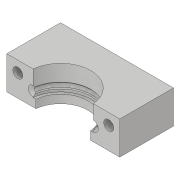
# Autodesk Inventor part: 7 peristaltic pump lid with lip2
Saved by Autodesk Inventor 2020 (Build 240168000, 168)
## iProperties
Created: 2018-08-21
Part Number: 7 peristaltic pump lid with lip2
Material: Generic
Document SubType Name: Modeling
Designer: mrbeh
Density: 1 g/cm^3
Appearance: Default
Author: mrbeh
Autodesk Inventor part; units mm, degrees
ref_plane "YZ Plane" through (0, 0, 0) normal (1, 0, 0) x (0, 1, 0)
ref_plane "XZ Plane" through (0, 0, 0) normal (0, 1, 0) x (-1, 0, 0)
sketch "Sketch1" plane through (0, 0, 0) normal (0, 1, 0) x (-1, 0, 0)
  line L0 (0, 0) -> (41, 0)
  line L1 (41, 0) -> (41, -41)
  line L2 (41, -41) -> (0, -41)
  line L3 (0, -41) -> (0, 0)
  dimension "d0" = 41
  dimension "d1" = 41
  constraints: 8 end point, 2 parallel, 1 horizontal, 1 perpendicular
  measures "d0" distance of L1.end L2.end
  measures "d1" distance of L0.end L1.end
extrude "Extrusion1" add sketch "Sketch1" along normal blind 9.5
sketch "Sketch3" plane through (0, 9.5, 0) normal (0, 1, 0) x (1, 0, 0)
  circle A0 centre (-20.5, 20.5) radius 10
  point P0 (0, 0)
  dimension "d5" = 20
  constraints: 1 centre point
  measures "d5" diameter of A0
extrude "Extrusion2" cut sketch "Sketch3" against normal blind 10
sketch "Sketch4" plane through (0, 9.5, 0) normal (0, 1, 0) x (1, 0, 0)
  circle A0 centre (-20.5, 20.5) radius 10 projected
  circle A1 centre (-20.5, 20.5) radius 11.75
  point P0 (0, 0)
  dimension "d8" = 23.5
  constraints: 1 centre point, 1 coincident
  measures "d8" diameter of A1
extrude "Extrusion3" cut sketch "Sketch4" against normal blind 5
sketch "Sketch5" plane through (0, 9.5, 0) normal (0, 1, 0) x (1, 0, 0)
  line L0 (-41, 41) -> (-41, 0) projected
  line L1 (-41, 0) -> (0, 0)
  line L2 (0, 0) -> (0, 41)
  line L3 (0, 41) -> (-41, 41)
  line L4 (-41, 41) -> (-41, 0)
  circle A0 centre (-20.5, 20.5) radius 11.75 projected
  circle A1 centre (-20.5, 20.5) radius 10
  constraints: 8 end point, 2 parallel, 1 centre point, 1 coincident, 1 horizontal, 1 perpendicular
extrude "Extrusion4" add sketch "Sketch5" along normal blind 4.5 contours L3 L2 L1 L0 | A0
sketch "Sketch6" plane through (-41, 0, 0) normal (0, 0, 1) x (1, 0, 0)
  line L0 (0, 0) -> (0, 14) projected
  line L1 (0, 14) -> (41, 14)
  line L2 (41, 14) -> (41, 0)
  line L3 (41, 0) -> (0, 0)
  line L4 (0, 0) -> (0, 14)
  constraints: 8 end point, 2 parallel, 1 horizontal, 1 perpendicular
extrude "Extrusion5" cut sketch "Sketch6" against normal blind 20.5
sketch "Sketch8" plane through (-41, 0, -20.5) normal (0, 0, 1) x (1, 0, 0)
  circle A0 centre (4, 10) radius 1.8
  point P0 (41, 0)
  dimension "d15" = 3.6
  constraints: 1 centre point
  measures "d15" diameter of A0
extrude "Extrusion6" cut sketch "Sketch8" against normal blind 20.5
ref_plane "Work Plane1" through (-20.5, 0, -41) normal (1, 0, 0) x (0, 0, -1)
mirror "Mirror1" about plane through (-20.5, 0, -41) normal (1, 0, 0) of "Extrusion6"
sketch "Sketch9" plane through (-41, 0, -20.5) normal (0, 0, 1) x (1, 0, 0)
  line L0 (10.5, 14) -> (10.5, 9.5) projected
  line L1 (8.75, 4.5) -> (10.5, 4.5) projected
  line L2 (10.5, 9.5) -> (8.75, 9.5)
  line L3 (8.75, 9.5) -> (8.75, 4.5)
  line L4 (8.75, 4.5) -> (10.5, 4.5)
  line L5 (10.5, 4.5) -> (10.5, 9.5)
  point P0 (41, 0)
  constraints: 8 end point, 2 parallel, 1 horizontal, 1 perpendicular
sketch "Sketch11" plane through (0, 4.5, 0) normal (0, 1, 0) x (1, 0, 0)
  arc A0 (-10.5, 20.5) -> (-30.5, 20.5) centre (-20.5, 20.5) ccw projected
  arc A1 (-9.625, 20.5) -> (-31.375, 20.5) centre (-20.5, 20.5) ccw
  line L0 (-41, 41) -> (-41, 20.5) projected
  point P0 (0, 0)
  constraints: 3 point on circle, 1 centre point, 1 coincident
sweep "Sweep1" add profiles "Sketch9" path "Sketch11" path curves A1
sketch "Sketch12" plane through (-41, 0, -20.5) normal (0, 0, 1) x (1, 0, 0)
  line L0 (10.5, 14) -> (10.5, 0) projected
  circle A0 centre (10.5, 7) radius 0.8
  point P0 (41, 0)
  dimension "d21" = 1.6
  constraints: 1 centre point, 1 midpoint
  measures "d21" diameter of A0
sketch3d "3D Sketch1"
  arc A0 (-30.5, 14, -20.5) -> (-27.5711, 14, -27.5711) centre (-20.5, 14, -20.5) ccw
  arc A1 (-27.5711, 14, -27.5711) -> (-20.5, 14, -30.5) centre (-20.5, 14, -20.5) ccw
  arc A2 (-20.5, 14, -30.5) -> (-13.4289, 14, -27.5711) centre (-20.5, 14, -20.5) ccw
  arc A3 (-13.4289, 14, -27.5711) -> (-10.5, 14, -20.5) centre (-20.5, 14, -20.5) ccw
sweep "Sweep2" cut profiles "Sketch12" path "3D Sketch1"
sketch "Sketch13" plane through (0, 0, 0) normal (0, -1, 0) x (1, 0, 0)
  line L0 (-53.975, -9.525) -> (46.0375, -9.525)
  line L1 (46.0375, -9.525) -> (46.0375, -71.4375)
  line L2 (46.0375, -71.4375) -> (-53.975, -71.4375)
  line L3 (-53.975, -71.4375) -> (-53.975, -9.525)
  point P0 (0, 0)
  constraints: 8 end point, 2 parallel, 1 horizontal, 1 perpendicular
extrude "Extrusion7" cut sketch "Sketch13" against normal blind 2
sketch "Sketch14" plane through (-41, 0, -20.5) normal (0, 0, 1) x (1, 0, 0)
  line L0 (-1.5875, 15.875) -> (46.0375, 15.875)
  line L1 (46.0375, 15.875) -> (46.0375, -1.5875)
  line L2 (46.0375, -1.5875) -> (-1.5875, -1.5875)
  line L3 (-1.5875, -1.5875) -> (-1.5875, 15.875)
  point P0 (41, 0)
  constraints: 8 end point, 2 parallel, 1 horizontal, 1 perpendicular
extrude "Extrusion8" cut sketch "Sketch14" against normal blind 0.7
sketch "Sketch15" plane through (0, 14, 0) normal (0, 1, 0) x (1, 0, 0)
  arc A0 (-10.5245, 21.2) -> (-30.4755, 21.2) centre (-20.5, 20.5) ccw projected
  circle A1 centre (-20.5, 20.5) radius 10.9575
  point P0 (0, 0)
  dimension "d28" = 21.915
  constraints: 1 centre point, 1 coincident
  measures "d28" diameter of A1
extrude "Extrusion9" cut sketch "Sketch15" against normal blind 15
sketch "Sketch16" plane through (-41, 0, -21.2) normal (0, 0, 1) x (1, 0, 0)
  line L0 (9.5649, 2) -> (9.5649, 14) projected
  circle A0 centre (9.5649, 7) radius 0.8
  point P0 (41, 0)
  dimension "d31" = 1.6
  constraints: 1 centre point, 1 point on line
  measures "d31" diameter of A0
sketch "Sketch17" plane through (0, 14, 0) normal (0, 1, 0) x (1, 0, 0)
  arc A0 (-9.5649, 21.2) -> (-31.4351, 21.2) centre (-20.5, 20.5) ccw projected
  arc A1 (-7.5073, 21.2) -> (-33.4927, 21.2) centre (-20.5, 20.5) ccw
  point P0 (0, 0)
  constraints: 2 point on circle, 1 centre point, 1 coincident
sketch3d "3D Sketch2"
  arc A0 (-31.4351, 14, -21.2) -> (-9.5649, 14, -21.2) centre (-20.5, 14, -20.5) ccw
sweep "Sweep3" cut profiles "Sketch16" path "3D Sketch2"
sketch "Sketch18" plane through (-41, 0, -21.2) normal (0, 0, 1) x (1, 0, 0)
  line L0 (31.4351, 7.8) -> (31.4351, 6.2) projected
  circle A0 centre (31.4351, 7) radius 0.8
  point P0 (41, 0)
  constraints: 1 midpoint, 1 vertical alignment, 2 other
sketch3d "3D Sketch3"
  arc A0 (-9.5649, 14, -21.2) -> (-31.4351, 14, -21.2) centre (-20.5, 14, -20.5) ccw
sweep "Sweep4" cut profiles "Sketch18" path "3D Sketch3"
sketch "Sketch19" plane through (-41, 0, -21.2) normal (0, 0, 1) x (1, 0, 0)
  line L0 (0, 2) -> (0, 14) projected
  line L1 (41, 2) -> (41, 14) projected
  line L2 (0, 14) -> (41, 14)
  line L3 (41, 14) -> (41, 2)
  line L4 (41, 2) -> (0, 2)
  line L5 (0, 2) -> (0, 14)
  point P0 (41, 0)
  constraints: 8 end point, 2 parallel, 1 horizontal, 1 perpendicular
extrude "Extrusion10" cut sketch "Sketch19" against normal blind 0.3
sketch "Sketch20" plane through (-41, 0, -21.5) normal (0, 0, 1) x (1, 0, 0)
  line L0 (9.5882, 6.2) -> (9.5882, 2) projected
  line L1 (9.5882, 2) -> (10.5882, 2)
  line L2 (10.5882, 2) -> (10.5882, 5)
  line L3 (10.5882, 5) -> (9.5882, 5)
  line L4 (9.5882, 5) -> (9.5882, 2)
  point P0 (41, 0)
  dimension "d38" = 1
  dimension "d39" = 3
  constraints: 8 end point, 2 parallel, 1 horizontal, 1 perpendicular
  measures "d38" distance of L3.end L2.end
  measures "d39" distance of L2.end L1.end
sweep "Sweep5" add profiles "Sketch20" path "Sketch17" path curves A0
sketch "Sketch21" plane through (-41, 0, -21.5) normal (0, 0, 1) x (1, 0, 0)
  line L0 (0, 2) -> (0, 14) projected
  line L1 (41, 2) -> (0, 2) projected
  line L2 (0, 14) -> (41, 14)
  line L3 (41, 14) -> (41, 2)
  line L4 (41, 2) -> (0, 2)
  line L5 (0, 2) -> (0, 14)
  point P0 (41, 0)
  constraints: 8 end point, 2 parallel, 1 horizontal, 1 perpendicular
extrude "Extrusion11" cut sketch "Sketch21" along normal blind 10
chamfer "Chamfer1" distance 1 angle 45 2 edges at (-8.7866, 7, -21.5) (-32.2134, 7, -21.5)
chamfer "Chamfer2" distance 0.3 angle 45 2 edges at (-20.4996, 7.8, -31.4575) (-20.4997, 6.2, -31.4575)
body "Solid1"
